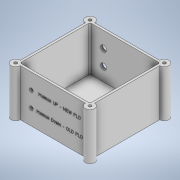
# Autodesk Inventor part: Case
Saved by Autodesk Inventor 2020 (Build 240168000, 168)
## iProperties
Created: 2019-12-06
Part Number: Case
Material: Generic
Document SubType Name: Modeling
Designer: Alex
Density: 1 g/cm^3
Appearance: Default
Author: Alex
Autodesk Inventor part; units mm, degrees
(part 1 of 2)
ref_plane "YZ Plane" through (0, 0, 0) normal (1, 0, 0) x (0, 1, 0)
ref_plane "XZ Plane" through (0, 0, 0) normal (0, 1, 0) x (-1, 0, 0)
ref_plane "XY Plane" through (0, 0, 0) normal (0, 0, 1) x (1, 0, 0)
sketch "Sketch1" plane through (0, 0, 0) normal (0, 1, 0) x (-1, 0, 0)
  line L0 (50, -50) -> (43.75, -50) construction
  line L1 (-50, -50) -> (-50, -43.75) construction
  line L2 (-50, 50) -> (-43.75, 50) construction
  line L3 (50, 50) -> (50, 43.75) construction
  arc A0 (43.75, -50) -> (50, -43.75) centre (50, -50) ccw
  arc A1 (-50, -43.75) -> (-43.75, -50) centre (-50, -50) ccw
  arc A2 (-43.75, 50) -> (-50, 43.75) centre (-50, 50) ccw
  arc A3 (50, 43.75) -> (43.75, 50) centre (50, 50) ccw
  line L4 (43.75, -50) -> (-43.75, -50)
  line L5 (50, -43.75) -> (50, -50) construction
  arc A4 (50, -43.75) -> (43.75, -50) centre (50, -50) ccw construction
  line L6 (50, 43.75) -> (50, -43.75)
  line L7 (43.75, 50) -> (50, 50) construction
  arc A5 (43.75, 50) -> (50, 43.75) centre (50, 50) ccw construction
  line L8 (-43.75, 50) -> (43.75, 50)
  line L9 (-50, 43.75) -> (-50, 50) construction
  arc A6 (-50, 43.75) -> (-43.75, 50) centre (-50, 50) ccw construction
  arc A7 (-43.75, -50) -> (-50, -43.75) centre (-50, -50) ccw construction
  line L10 (-43.75, -50) -> (-50, -50) construction
  line L11 (-50, -43.75) -> (-50, 43.75)
  point P0 (0, 0)
  point P1 (50, 0)
  point P2 (0, -50)
  dimension "d0" = 100
  dimension "d1" = 100
  dimension "d3" = 6.25
  constraints: 24 end point, 18 parallel, 16 point on circle, 9 perpendicular, 8 centre point, 4 coincident, 3 equal radius, 3 horizontal, 2 midpoint, 1 horizontal alignment, 1 vertical alignment
  measures "d0" distance of L1.start L0.start
  measures "d1" distance of L2.start L1.start
  measures "d3" radius of A0
extrude "Extrusion1" add sketch "Sketch1" along normal blind 3
sketch "Sketch2" plane through (0, 3, 0) normal (0, 1, 0) x (1, 0, 0)
  arc A0 (50, 43.75) -> (43.75, 50) centre (50, 50) ccw projected
  line L0 (43.75, 50) -> (-43.75, 50) projected
  arc A1 (-43.75, 50) -> (-50, 43.75) centre (-50, 50) ccw projected
  line L1 (-50, 43.75) -> (-50, -43.75) projected
  arc A2 (-50, -43.75) -> (-43.75, -50) centre (-50, -50) ccw projected
  line L2 (-43.75, -50) -> (43.75, -50) projected
  arc A3 (43.75, -50) -> (50, -43.75) centre (50, -50) ccw projected
  line L3 (50, -43.75) -> (50, 43.75) projected
  line L4 (-45, 47) -> (45, 47)
  line L5 (47, 45) -> (47, -45)
  line L6 (45, -47) -> (-45, -47)
  line L7 (-47, -45) -> (-47, 45)
  arc A4 (-45, 47) -> (-47, 45) centre (-45, 45) ccw
  arc A5 (-47, -45) -> (-45, -47) centre (-45, -45) ccw
  arc A6 (45, -47) -> (47, -45) centre (45, -45) ccw
  arc A7 (47, 45) -> (45, 47) centre (45, 45) ccw
  point P0 (0, 0)
  dimension "d6" = 3
  dimension "d7" = 2
  constraints: 8 end point, 8 point on circle, 8 tangent, 4 centre point, 3 equal radius, 3 other
  measures "d6" distance between parallel lines of L0 L4
  measures "d7" radius of A4
extrude "Extrusion2" add sketch "Sketch2" along normal blind 60
sketch "Sketch3" plane through (0, 63, 0) normal (0, 1, 0) x (1, 0, 0)
  arc A0 (-50, -43.75) -> (-43.75, -50) centre (-50, -50) ccw construction
  line L0 (-43.75, -50) -> (43.75, -50) construction
  arc A1 (43.75, -50) -> (50, -43.75) centre (50, -50) ccw construction
  line L1 (50, -43.75) -> (50, 43.75) construction
  arc A2 (50, 43.75) -> (43.75, 50) centre (50, 50) ccw construction
  line L2 (43.75, 50) -> (-43.75, 50) construction
  arc A3 (-43.75, 50) -> (-50, 43.75) centre (-50, 50) ccw construction
  line L3 (-50, 43.75) -> (-50, -43.75) construction
  line L4 (-45, 47) -> (45, 47) construction
  arc A4 (47, 45) -> (45, 47) centre (45, 45) ccw construction
  line L5 (47, 45) -> (47, -45) construction
  arc A5 (45, -47) -> (47, -45) centre (45, -45) ccw construction
  line L6 (45, -47) -> (-45, -47) construction
  arc A6 (-47, -45) -> (-45, -47) centre (-45, -45) ccw construction
  line L7 (-47, -45) -> (-47, 45) construction
  arc A7 (-45, 47) -> (-47, 45) centre (-45, 45) ccw construction
  point P0 (0, 0)
  constraints: 4 coincident
hole "Hole1" at (-50, 63, -50) at (50, 63, -50) at (50, 63, 50) at (-50, 63, 50) direction (0, -1, 0) diameter 4 depth 5
sketch "Sketch4" plane through (0, 3, 0) normal (0, 1, 0) x (1, 0, 0)
  line L0 (-9.3, 44) -> (44, 44) construction
  line L1 (44, 44) -> (44, -24.6) construction
  line L2 (44, -24.6) -> (-9.3, -24.6) construction
  line L3 (-9.3, -24.6) -> (-9.3, 44) construction
  arc A0 (-45, 47) -> (-47, 45) centre (-45, 45) ccw construction
  line L4 (-47, 45) -> (-47, -45) construction
  arc A1 (-47, -45) -> (-45, -47) centre (-45, -45) ccw construction
  line L5 (-45, -47) -> (45, -47) construction
  arc A2 (45, -47) -> (47, -45) centre (45, -45) ccw construction
  line L6 (47, -45) -> (47, 45) construction
  arc A3 (47, 45) -> (45, 47) centre (45, 45) ccw construction
  line L7 (45, 47) -> (-45, 47) construction
  line L8 (-4.2, -24.6) -> (0.8, -24.6)
  line L9 (0.8, -24.6) -> (0.8, -19.6)
  line L10 (0.8, -19.6) -> (-4.2, -19.6)
  line L11 (-4.2, -19.6) -> (-4.2, -24.6)
  line L12 (-4.2, -24.6) -> (0.8, -19.6) construction
  line L13 (0.8, -24.6) -> (-4.2, -19.6) construction
  line L14 (28.7, -24.6) -> (23.7, -24.6)
  line L15 (23.7, -24.6) -> (23.7, -19.6)
  line L16 (23.7, -19.6) -> (28.7, -19.6)
  line L17 (28.7, -19.6) -> (28.7, -24.6)
  line L18 (28.7, -24.6) -> (23.7, -19.6) construction
  line L19 (23.7, -24.6) -> (28.7, -19.6) construction
  line L20 (-8.3, 29) -> (13.7, 29)
  line L21 (13.7, 29) -> (13.7, 19)
  line L22 (13.7, 19) -> (-8.3, 19)
  line L23 (-8.3, 19) -> (-8.3, 29)
  line L24 (33, 37) -> (43, 37)
  line L25 (43, 37) -> (43, 32)
  line L26 (43, 32) -> (33, 32)
  line L27 (33, 32) -> (33, 37)
  point P0 (0, 0)
  point P1 (-6.8, 30)
  point P2 (41.4, 28.7)
  point P3 (-1.7, -22.1)
  point P4 (26.2, -22.1)
  dimension "d17" = 68.6
  dimension "d18" = 53.3
  dimension "d19" = 14
  dimension "d20" = 1.3
  dimension "d21" = 50.8
  dimension "d22" = 2.5
  dimension "d23" = 5.1
  dimension "d24" = 27.9
  dimension "d25" = 15.2
  dimension "d26" = 3
  dimension "d27" = 3
  dimension "d28" = 5
  dimension "d29" = 15
  dimension "d30" = 25
  dimension "d31" = 1
  dimension "d32" = 23
  dimension "d33" = 7
  dimension "d34" = 12
  dimension "d35" = 1
  dimension "d36" = 11
  constraints: 48 end point, 10 parallel, 5 horizontal, 5 perpendicular, 4 midpoint, 3 equal length, 1 horizontal alignment
  measures "d17" distance of L2.end L0.start
  measures "d18" distance of L0.start L0.end
  measures "d19" distance from line of point (-6.8, 30) L0
  measures "d20" vertical distance of point (41.4, 28.7) point (-6.8, 30)
  measures "d21" vertical distance of point (26.2, -22.1) point (41.4, 28.7)
  measures "d22" distance from line of point (-6.8, 30) L3
  measures "d23" horizontal distance of point (-1.7, -22.1) point (-6.8, 30)
  measures "d24" distance of point (26.2, -22.1) point (-1.7, -22.1)
  measures "d25" horizontal distance of point (41.4, 28.7) point (26.2, -22.1)
  measures "d26" distance between parallel lines of L0 L7
  measures "d27" distance between parallel lines of L6 L1
  measures "d28" distance of L9.end L10.end
  measures "d29" distance between parallel lines of L20 L0
  measures "d30" distance between parallel lines of L22 L0
  measures "d31" distance between parallel lines of L23 L3
  measures "d32" distance between parallel lines of L21 L3
  measures "d33" distance between parallel lines of L24 L0
  measures "d34" distance between parallel lines of L26 L0
  measures "d35" distance between parallel lines of L25 L1
  measures "d36" distance between parallel lines of L27 L1
extrude "Extrusion3" add sketch "Sketch4" along normal blind 3
chamfer "Chamfer1" distance 3 angle 45 16 edges at (2.7, 3, -19) (-8.3, 3, -24) (2.7, 3, -29) (13.7, 3, -24) (38, 3, -32) (33, 3, -34.5) (43, 3, -34.5) (38, 3, -37) (-4.2, 3, 22.1) (-1.7, 3, 19.6) (-1.7, 3, 24.6) (0.8, 3, 22.1) (26.2, 3, 24.6) (28.7, 3, 22.1) (23.7, 3, 22.1) (26.2, 3, 19.6)
sketch "Sketch5" plane through (0, 6, 0) normal (0, 1, 0) x (1, 0, 0)
  line L0 (0.8, -19.6) -> (-4.2, -19.6) projected
  line L1 (28.7, -19.6) -> (23.7, -19.6) projected
  line L2 (0.8, -24.6) -> (0.8, -19.6) projected
  point P0 (0, 0)
  point P1 (-1.7, -22.1)
  point P2 (26.2, -22.1)
  point P3 (-1.7, -19.6)
  point P4 (26.2, -19.6)
  point P5 (0.8, -22.1)
  point P6 (0.8, -22.1)
  constraints: 4 midpoint, 2 horizontal alignment, 2 vertical alignment
hole "Hole2" at (-1.7, 6, 22.1) at (26.2, 6, 22.1) direction (0, -1, 0) diameter 4 depth 5
sketch "Sketch6" plane through (-45, 3, -47) normal (0, 0, 1) x (1, 0, 0)
  line L0 (67.7, 15.6) -> (79.9, 15.6)
  line L1 (79.9, 15.6) -> (79.9, 4.6)
  line L2 (79.9, 4.6) -> (67.7, 4.6)
  line L3 (67.7, 4.6) -> (67.7, 15.6)
  line L4 (36.7, 3) -> (58.7, 3) construction
  line L5 (58.7, 3) -> (36.7, 3) construction
  line L6 (33.7, 0) -> (61.7, 0) construction
  line L7 (58.7, 3) -> (61.7, 0) construction
  line L8 (36.7, 3) -> (58.7, 3) construction
  line L9 (33.7, 0) -> (36.7, 3) construction
  line L10 (33.7, 0) -> (36.7, 3) construction
  line L11 (36.7, 3) -> (33.7, 0) construction
  line L12 (58.7, 3) -> (61.7, 0) construction
  line L13 (58.7, 3) -> (61.7, 0) construction
  line L14 (61.7, 0) -> (33.7, 0) construction
  line L15 (36.7, 3) -> (33.7, 0) construction
  line L16 (58.7, 3) -> (36.7, 3) construction
  line L17 (58.7, 3) -> (61.7, 0) construction
  point P0 (45, -3)
  point P1 (35.7, 0)
  point P2 (35.7, 0)
  point P3 (35.7, 0)
  point P4 (89, 0)
  point P5 (89, 0)
  point P6 (89, 0)
  dimension "d49" = 1.6
  dimension "d50" = 12.2
  dimension "d51" = 11
  dimension "d52" = 9.1
  constraints: 8 end point, 2 parallel, 1 horizontal, 1 perpendicular
  measures "d49" distance between parallel lines of L4 L2
  measures "d50" distance of L0.start L0.end
  measures "d51" distance of L2.end L0.start
  measures "d52" distance from line of L1 point (89, 0)
extrude "Extrusion4" cut sketch "Sketch6" against normal blind 3
sketch "Sketch7" plane through (43.75, 0, -50) normal (0, 0, -1) x (-1, 0, 0)
  line L0 (72.5, 42) -> (72.5, 63) construction
  line L1 (87.5, 63) -> (0, 63) construction
  line L2 (21.05, 7.6) -> (8.85, 7.6) construction
  line L3 (8.85, 7.6) -> (8.85, 18.6) construction
  line L4 (8.85, 18.6) -> (21.05, 18.6) construction
  line L5 (21.05, 18.6) -> (21.05, 7.6) construction
  line L6 (0, 0) -> (87.5, 0) construction
  line L7 (87.5, 0) -> (87.5, 63) construction
  line L8 (0, 63) -> (87.5, 63) construction
  line L9 (0, 0) -> (0, 63) construction
  line L10 (72.5, 42) -> (72.5, 21) construction
  line L11 (72.5, 21) -> (72.5, 0) construction
  line L12 (87.5, 0) -> (0, 0) construction
  point P0 (43.75, 0)
  dimension "d55" = 15
  constraints: 6 end point, 3 point on line, 2 collinear, 2 vertical, 1 vertical alignment
  measures "d55" distance between parallel lines of L7 L10
hole "Hole3" at (-28.75, 42, -50) at (-28.75, 21, -50) direction (0, 0, 1) diameter 8 depth 5
sketch "Sketch8" plane through (-43.75, 0, 50) normal (0, 0, 1) x (1, 0, 0)
  line L0 (0, 0) -> (87.5, 0) construction
  line L1 (87.5, 0) -> (87.5, 63) construction
  line L2 (0, 63) -> (87.5, 63) construction
  line L3 (0, 0) -> (0, 63) construction
  line L4 (15, 42) -> (15, 63) construction
  line L5 (15, 21) -> (15, 0) construction
  line L6 (87.5, 0) -> (0, 0) construction
  line L7 (15, 42) -> (15, 21) construction
  point P0 (43.75, 0)
  dimension "d63" = 15
  constraints: 6 end point, 3 vertical, 2 collinear, 2 point on line
  measures "d63" distance between parallel lines of L4 L3
hole "Hole4" at (-28.75, 42, 50) at (-28.75, 21, 50) direction (0, 0, -1) diameter 5 depth 5
sketch "Sketch9" plane through (-43.75, 0, 50) normal (0, 0, 1) x (1, 0, 0)
  line L0 (20.5, 47) -> (85.5, 47) construction
  line L1 (85.5, 47) -> (85.5, 37) construction
  line L2 (85.5, 37) -> (20.5, 37) construction
  line L3 (20.5, 37) -> (20.5, 47) construction
  line L4 (20.5, 26) -> (85.5, 26) construction
  line L5 (85.5, 26) -> (85.5, 16) construction
  line L6 (85.5, 16) -> (20.5, 16) construction
  line L7 (20.5, 16) -> (20.5, 26) construction
  circle A0 centre (15, 42) radius 2.5 construction
  circle A1 centre (15, 21) radius 2.5 construction
  line L8 (0, 0) -> (87.5, 0) construction
  line L9 (87.5, 0) -> (87.5, 63) construction
  line L10 (0, 63) -> (87.5, 63) construction
  line L11 (0, 0) -> (0, 63) construction
  spline S0 degree 2 poles (28.025, 40.2168) (28.025, 40.0318) (27.8491, 40.0318) knots 0 0 0 1 1 1
  spline S1 degree 2 poles (27.8491, 40.0318) (27.6702, 40.0318) (27.6702, 40.2168) knots 0 0 0 1 1 1
  line L12 (27.6702, 40.2168) -> (27.6702, 43.3859)
  line L13 (27.6702, 43.3859) -> (26.627, 41.8757)
  spline S2 degree 2 poles (26.627, 41.8757) (26.533, 41.7422) (26.4117, 41.7422) knots 0 0 0 1 1 1
  spline S3 degree 2 poles (26.4117, 41.7422) (26.2964, 41.7422) (26.2146, 41.8605) knots 0 0 0 1 1 1
  line L14 (26.2146, 41.8605) -> (25.1713, 43.398)
  line L15 (25.1713, 43.398) -> (25.1713, 40.2168)
  spline S4 degree 2 poles (25.1713, 40.2168) (25.1713, 40.0318) (24.9924, 40.0318) knots 0 0 0 1 1 1
  spline S5 degree 2 poles (24.9924, 40.0318) (24.8105, 40.0318) (24.8105, 40.2168) knots 0 0 0 1 1 1
  line L16 (24.8105, 40.2168) -> (24.8105, 43.8105)
  spline S6 degree 2 poles (24.8105, 43.8105) (24.8105, 44.0076) (25.0076, 44.0076) knots 0 0 0 1 1 1
  spline S7 degree 2 poles (25.0076, 44.0076) (25.1744, 44.0076) (25.2866, 43.8499) knots 0 0 0 1 1 1
  line L17 (25.2866, 43.8499) -> (26.4177, 42.2244)
  line L18 (26.4177, 42.2244) -> (27.5519, 43.8469)
  spline S8 degree 2 poles (27.5519, 43.8469) (27.6823, 44.0318) (27.834, 44.0318) knots 0 0 0 1 1 1
  spline S9 degree 2 poles (27.834, 44.0318) (28.025, 44.0318) (28.025, 43.8105) knots 0 0 0 1 1 1
  line L19 (28.025, 43.8105) -> (28.025, 40.2168)
  spline S10 degree 2 poles (29.514, 40.2229) (29.514, 40.0379) (29.3351, 40.0379) knots 0 0 0 1 1 1
  spline S11 degree 2 poles (29.3351, 40.0379) (29.1531, 40.0379) (29.1531, 40.2229) knots 0 0 0 1 1 1
  line L20 (29.1531, 40.2229) -> (29.1531, 43.119)
  spline S12 degree 2 poles (29.1531, 43.119) (29.1531, 43.304) (29.3351, 43.304) knots 0 0 0 1 1 1
  spline S13 degree 2 poles (29.3351, 43.304) (29.514, 43.304) (29.514, 43.119) knots 0 0 0 1 1 1
  line L21 (29.514, 43.119) -> (29.514, 40.2229)
  spline S14 degree 2 poles (32.7559, 42.4003) (32.7559, 41.9181) (32.4375, 41.6725) knots 0 0 0 1 1 1
  spline S15 degree 2 poles (32.4375, 41.6725) (32.2252, 41.5057) (32.0159, 41.5057) knots 0 0 0 1 1 1
  line L22 (32.0159, 41.5057) -> (31.9219, 41.5087)
  line L23 (31.9219, 41.5087) -> (32.7225, 40.323)
  spline S16 degree 2 poles (32.7225, 40.323) (32.7559, 40.2684) (32.7559, 40.2168) knots 0 0 0 1 1 1
  spline S17 degree 2 poles (32.7559, 40.2168) (32.7559, 40.141) (32.6467, 40.0318) (32.577, 40.0318) knots 0 0 0 1 2 2 2
  spline S18 degree 2 poles (32.577, 40.0318) (32.4951, 40.0318) (32.4435, 40.1077) knots 0 0 0 1 1 1
  line L24 (32.4435, 40.1077) -> (31.4913, 41.5057)
  line L25 (31.4913, 41.5057) -> (30.8241, 41.5057)
  line L26 (30.8241, 41.5057) -> (30.8241, 40.2168)
  spline S19 degree 2 poles (30.8241, 40.2168) (30.8241, 40.0318) (30.6513, 40.0318) knots 0 0 0 1 1 1
  spline S20 degree 2 poles (30.6513, 40.0318) (30.4754, 40.0318) (30.4754, 40.2168) knots 0 0 0 1 1 1
  line L27 (30.4754, 40.2168) -> (30.4754, 43.298)
  line L28 (30.4754, 43.298) -> (31.84, 43.298)
  spline S21 degree 2 poles (31.84, 43.298) (32.2221, 43.298) (32.4769, 43.0705) knots 0 0 0 1 1 1
  spline S22 degree 2 poles (32.4769, 43.0705) (32.7559, 42.8218) (32.7559, 42.4003) knots 0 0 0 1 1 1
  spline S23 degree 2 poles (32.4071, 42.4003) (32.4071, 42.6581) (32.0766, 42.9371) (31.84, 42.9371) knots 0 0 0 1 2 2 2
  line L29 (31.84, 42.9371) -> (30.8241, 42.9371)
  line L30 (30.8241, 42.9371) -> (30.8241, 41.8666)
  line L31 (30.8241, 41.8666) -> (32.0129, 41.8666)
  spline S24 degree 2 poles (32.0129, 41.8666) (32.1221, 41.8666) (32.2434, 41.9757) knots 0 0 0 1 1 1
  spline S25 degree 2 poles (32.2434, 41.9757) (32.4071, 42.1274) (32.4071, 42.4003) knots 0 0 0 1 1 1
  spline S26 degree 2 poles (35.6187, 42.4003) (35.6187, 41.9181) (35.3002, 41.6725) knots 0 0 0 1 1 1
  spline S27 degree 2 poles (35.3002, 41.6725) (35.0879, 41.5057) (34.8787, 41.5057) knots 0 0 0 1 1 1
  line L32 (34.8787, 41.5057) -> (34.7847, 41.5087)
  line L33 (34.7847, 41.5087) -> (35.5853, 40.323)
  spline S28 degree 2 poles (35.5853, 40.323) (35.6187, 40.2684) (35.6187, 40.2168) knots 0 0 0 1 1 1
  spline S29 degree 2 poles (35.6187, 40.2168) (35.6187, 40.141) (35.5095, 40.0318) (35.4397, 40.0318) knots 0 0 0 1 2 2 2
  spline S30 degree 2 poles (35.4397, 40.0318) (35.3578, 40.0318) (35.3063, 40.1077) knots 0 0 0 1 1 1
  line L34 (35.3063, 40.1077) -> (34.3541, 41.5057)
  line L35 (34.3541, 41.5057) -> (33.6869, 41.5057)
  line L36 (33.6869, 41.5057) -> (33.6869, 40.2168)
  spline S31 degree 2 poles (33.6869, 40.2168) (33.6869, 40.0318) (33.514, 40.0318) knots 0 0 0 1 1 1
  spline S32 degree 2 poles (33.514, 40.0318) (33.3381, 40.0318) (33.3381, 40.2168) knots 0 0 0 1 1 1
  line L37 (33.3381, 40.2168) -> (33.3381, 43.298)
  line L38 (33.3381, 43.298) -> (34.7028, 43.298)
  spline S33 degree 2 poles (34.7028, 43.298) (35.0849, 43.298) (35.3397, 43.0705) knots 0 0 0 1 1 1
  spline S34 degree 2 poles (35.3397, 43.0705) (35.6187, 42.8218) (35.6187, 42.4003) knots 0 0 0 1 1 1
  spline S35 degree 2 poles (35.2699, 42.4003) (35.2699, 42.6581) (34.9393, 42.9371) (34.7028, 42.9371) knots 0 0 0 1 2 2 2
  line L39 (34.7028, 42.9371) -> (33.6869, 42.9371)
  line L40 (33.6869, 42.9371) -> (33.6869, 41.8666)
  line L41 (33.6869, 41.8666) -> (34.8757, 41.8666)
  spline S36 degree 2 poles (34.8757, 41.8666) (34.9848, 41.8666) (35.1061, 41.9757) knots 0 0 0 1 1 1
  spline S37 degree 2 poles (35.1061, 41.9757) (35.2699, 42.1274) (35.2699, 42.4003) knots 0 0 0 1 1 1
  spline S38 degree 2 poles (38.5299, 41.6694) (38.5299, 41.0296) (38.2115, 40.5534) knots 0 0 0 1 1 1
  spline S39 degree 2 poles (38.2115, 40.5534) (37.8628, 40.0379) (37.323, 40.0379) knots 0 0 0 1 1 1
  spline S40 degree 2 poles (37.323, 40.0379) (36.7832, 40.0379) (36.4344, 40.5595) knots 0 0 0 1 1 1
  spline S41 degree 2 poles (36.4344, 40.5595) (36.116, 41.0356) (36.116, 41.6694) knots 0 0 0 1 1 1
  spline S42 degree 2 poles (36.116, 41.6694) (36.116, 42.2972) (36.4405, 42.7794) knots 0 0 0 1 1 1
  spline S43 degree 2 poles (36.4405, 42.7794) (36.7953, 43.2889) (37.323, 43.2889) knots 0 0 0 1 1 1
  spline S44 degree 2 poles (37.323, 43.2889) (37.887, 43.2889) (38.2237, 42.7733) knots 0 0 0 1 1 1
  spline S45 degree 2 poles (38.2237, 42.7733) (38.5299, 42.3063) (38.5299, 41.6694) knots 0 0 0 1 1 1
  spline S46 degree 2 poles (38.1812, 41.6694) (38.1812, 42.1668) (37.978, 42.5155) knots 0 0 0 1 1 1
  spline S47 degree 2 poles (37.978, 42.5155) (37.7475, 42.928) (37.323, 42.928) knots 0 0 0 1 1 1
  spline S48 degree 2 poles (37.323, 42.928) (36.9227, 42.928) (36.6801, 42.5155) knots 0 0 0 1 1 1
  spline S49 degree 2 poles (36.6801, 42.5155) (36.4647, 42.1577) (36.4647, 41.6694) knots 0 0 0 1 1 1
  spline S50 degree 2 poles (36.4647, 41.6694) (36.4647, 41.1691) (36.674, 40.8112) knots 0 0 0 1 1 1
  spline S51 degree 2 poles (36.674, 40.8112) (36.9105, 40.3988) (37.323, 40.3988) knots 0 0 0 1 1 1
  spline S52 degree 2 poles (37.323, 40.3988) (37.7354, 40.3988) (37.9719, 40.8112) knots 0 0 0 1 1 1
  spline S53 degree 2 poles (37.9719, 40.8112) (38.1812, 41.1691) (38.1812, 41.6694) knots 0 0 0 1 1 1
  spline S54 degree 2 poles (41.4473, 42.4003) (41.4473, 41.9181) (41.1289, 41.6725) knots 0 0 0 1 1 1
  spline S55 degree 2 poles (41.1289, 41.6725) (40.9166, 41.5057) (40.7074, 41.5057) knots 0 0 0 1 1 1
  line L42 (40.7074, 41.5057) -> (40.6133, 41.5087)
  line L43 (40.6133, 41.5087) -> (41.414, 40.323)
  spline S56 degree 2 poles (41.414, 40.323) (41.4473, 40.2684) (41.4473, 40.2168) knots 0 0 0 1 1 1
  spline S57 degree 2 poles (41.4473, 40.2168) (41.4473, 40.141) (41.3381, 40.0318) (41.2684, 40.0318) knots 0 0 0 1 2 2 2
  spline S58 degree 2 poles (41.2684, 40.0318) (41.1865, 40.0318) (41.135, 40.1077) knots 0 0 0 1 1 1
  line L44 (41.135, 40.1077) -> (40.1827, 41.5057)
  line L45 (40.1827, 41.5057) -> (39.5155, 41.5057)
  line L46 (39.5155, 41.5057) -> (39.5155, 40.2168)
  spline S59 degree 2 poles (39.5155, 40.2168) (39.5155, 40.0318) (39.3427, 40.0318) knots 0 0 0 1 1 1
  spline S60 degree 2 poles (39.3427, 40.0318) (39.1668, 40.0318) (39.1668, 40.2168) knots 0 0 0 1 1 1
  line L47 (39.1668, 40.2168) -> (39.1668, 43.298)
  line L48 (39.1668, 43.298) -> (40.5315, 43.298)
  spline S61 degree 2 poles (40.5315, 43.298) (40.9136, 43.298) (41.1683, 43.0705) knots 0 0 0 1 1 1
  spline S62 degree 2 poles (41.1683, 43.0705) (41.4473, 42.8218) (41.4473, 42.4003) knots 0 0 0 1 1 1
  spline S63 degree 2 poles (41.0986, 42.4003) (41.0986, 42.6581) (40.768, 42.9371) (40.5315, 42.9371) knots 0 0 0 1 2 2 2
  line L49 (40.5315, 42.9371) -> (39.5155, 42.9371)
  line L50 (39.5155, 42.9371) -> (39.5155, 41.8666)
  line L51 (39.5155, 41.8666) -> (40.7043, 41.8666)
  spline S64 degree 2 poles (40.7043, 41.8666) (40.8135, 41.8666) (40.9348, 41.9757) knots 0 0 0 1 1 1
  spline S65 degree 2 poles (40.9348, 41.9757) (41.0986, 42.1274) (41.0986, 42.4003) knots 0 0 0 1 1 1
  spline S66 degree 2 poles (47.0455, 41.3419) (47.0455, 40.1077) (45.7354, 40.0076) knots 0 0 0 1 1 1
  spline S67 degree 2 poles (45.7354, 40.0076) (45.1895, 39.9682) (44.765, 40.2926) knots 0 0 0 1 1 1
  spline S68 degree 2 poles (44.765, 40.2926) (44.2889, 40.6626) (44.2889, 41.3086) knots 0 0 0 1 1 1
  line L52 (44.2889, 41.3086) -> (44.2889, 43.8408)
  spline S69 degree 2 poles (44.2889, 43.8408) (44.2889, 44.0258) (44.4678, 44.0258) knots 0 0 0 1 1 1
  spline S70 degree 2 poles (44.4678, 44.0258) (44.6437, 44.0258) (44.6437, 43.8408) knots 0 0 0 1 1 1
  line L53 (44.6437, 43.8408) -> (44.6437, 41.3086)
  spline S71 degree 2 poles (44.6437, 41.3086) (44.6437, 40.8446) (44.9985, 40.5716) knots 0 0 0 1 1 1
  spline S72 degree 2 poles (44.9985, 40.5716) (45.3108, 40.3321) (45.7111, 40.3624) knots 0 0 0 1 1 1
  spline S73 degree 2 poles (45.7111, 40.3624) (46.6907, 40.4261) (46.6907, 41.345) knots 0 0 0 1 1 1
  line L54 (46.6907, 41.345) -> (46.6907, 43.8408)
  spline S74 degree 2 poles (46.6907, 43.8408) (46.6907, 44.0258) (46.8696, 44.0258) knots 0 0 0 1 1 1
  spline S75 degree 2 poles (46.8696, 44.0258) (47.0455, 44.0258) (47.0455, 43.8408) knots 0 0 0 1 1 1
  line L55 (47.0455, 43.8408) -> (47.0455, 41.3419)
  spline S76 degree 2 poles (50.257, 42.9917) (50.257, 42.5489) (50.0235, 42.2881) knots 0 0 0 1 1 1
  spline S77 degree 2 poles (50.0235, 42.2881) (49.7809, 42.0091) (49.3442, 42.0091) knots 0 0 0 1 1 1
  line L56 (49.3442, 42.0091) -> (48.0796, 42.0091)
  line L57 (48.0796, 42.0091) -> (48.0796, 40.2168)
  spline S78 degree 2 poles (48.0796, 40.2168) (48.0796, 40.0318) (47.9037, 40.0318) knots 0 0 0 1 1 1
  spline S79 degree 2 poles (47.9037, 40.0318) (47.7248, 40.0318) (47.7248, 40.2168) knots 0 0 0 1 1 1
  line L58 (47.7248, 40.2168) -> (47.7248, 44.0197)
  line L59 (47.7248, 44.0197) -> (49.2472, 44.0197)
  spline S80 degree 2 poles (49.2472, 44.0197) (49.7566, 44.0197) (50.0174, 43.7286) knots 0 0 0 1 1 1
  spline S81 degree 2 poles (50.0174, 43.7286) (50.257, 43.4617) (50.257, 42.9917) knots 0 0 0 1 1 1
  spline S82 degree 2 poles (49.9022, 42.9917) (49.9022, 43.6588) (49.2472, 43.6588) knots 0 0 0 1 1 1
  line L60 (49.2472, 43.6588) -> (48.0796, 43.6588)
  line L61 (48.0796, 43.6588) -> (48.0796, 42.376)
  line L62 (48.0796, 42.376) -> (49.3442, 42.376)
  spline S83 degree 2 poles (49.3442, 42.376) (49.6111, 42.376) (49.9022, 42.7127) (49.9022, 42.9917) knots 0 0 0 1 2 2 2
  line L63 (54.7968, 41.4996) -> (53.3563, 41.4996)
  spline S84 degree 2 poles (53.3563, 41.4996) (53.1774, 41.4996) (53.1774, 41.6785) knots 0 0 0 1 1 1
  spline S85 degree 2 poles (53.1774, 41.6785) (53.1774, 41.8544) (53.3563, 41.8544) knots 0 0 0 1 1 1
  line L64 (53.3563, 41.8544) -> (54.7968, 41.8544)
  spline S86 degree 2 poles (54.7968, 41.8544) (54.9757, 41.8544) (54.9757, 41.6785) knots 0 0 0 1 1 1
  spline S87 degree 2 poles (54.9757, 41.6785) (54.9757, 41.4996) (54.7968, 41.4996) knots 0 0 0 1 1 1
  spline S88 degree 2 poles (60.7346, 40.2077) (60.7346, 40.0318) (60.5951, 40.0318) knots 0 0 0 1 1 1
  spline S89 degree 2 poles (60.5951, 40.0318) (60.4829, 40.0318) (60.3889, 40.1622) knots 0 0 0 1 1 1
  line L65 (60.3889, 40.1622) -> (58.2115, 43.3071)
  line L66 (58.2115, 43.3071) -> (58.2115, 40.2168)
  spline S90 degree 2 poles (58.2115, 40.2168) (58.2115, 40.0318) (58.0326, 40.0318) knots 0 0 0 1 1 1
  spline S91 degree 2 poles (58.0326, 40.0318) (57.8506, 40.0318) (57.8506, 40.2168) knots 0 0 0 1 1 1
  line L67 (57.8506, 40.2168) -> (57.8506, 43.862)
  spline S92 degree 2 poles (57.8506, 43.862) (57.8506, 44.0318) (58.0083, 44.0318) knots 0 0 0 1 1 1
  spline S93 degree 2 poles (58.0083, 44.0318) (58.1296, 44.0318) (58.2237, 43.8984) knots 0 0 0 1 1 1
  line L68 (58.2237, 43.8984) -> (60.3798, 40.8021)
  line L69 (60.3798, 40.8021) -> (60.3798, 43.8469)
  spline S94 degree 2 poles (60.3798, 43.8469) (60.3798, 44.0318) (60.5588, 44.0318) knots 0 0 0 1 1 1
  spline S95 degree 2 poles (60.5588, 44.0318) (60.7346, 44.0318) (60.7346, 43.8469) knots 0 0 0 1 1 1
  line L70 (60.7346, 43.8469) -> (60.7346, 40.2077)
  line L71 (64.0159, 40.0895) -> (61.5838, 40.0895)
  line L72 (61.5838, 40.0895) -> (61.5838, 44.0197)
  line L73 (61.5838, 44.0197) -> (64.0159, 44.0197)
  spline S96 degree 2 poles (64.0159, 44.0197) (64.1948, 44.0197) (64.1948, 43.8378) knots 0 0 0 1 1 1
  spline S97 degree 2 poles (64.1948, 43.8378) (64.1948, 43.6528) (64.0159, 43.6528) knots 0 0 0 1 1 1
  line L74 (64.0159, 43.6528) -> (61.9386, 43.6528)
  line L75 (61.9386, 43.6528) -> (61.9386, 42.4276)
  line L76 (61.9386, 42.4276) -> (63.8946, 42.4276)
  spline S98 degree 2 poles (63.8946, 42.4276) (64.0796, 42.4276) (64.0796, 42.2487) knots 0 0 0 1 1 1
  spline S99 degree 2 poles (64.0796, 42.2487) (64.0796, 42.0667) (63.8946, 42.0667) knots 0 0 0 1 1 1
  line L77 (63.8946, 42.0667) -> (61.9386, 42.0667)
  line L78 (61.9386, 42.0667) -> (61.9386, 40.4503)
  line L79 (61.9386, 40.4503) -> (64.0159, 40.4503)
  spline S100 degree 2 poles (64.0159, 40.4503) (64.1948, 40.4503) (64.1948, 40.2714) knots 0 0 0 1 1 1
  spline S101 degree 2 poles (64.1948, 40.2714) (64.1948, 40.0895) (64.0159, 40.0895) knots 0 0 0 1 1 1
  line L80 (68.9257, 43.8044) -> (68.2312, 40.2047)
  spline S102 degree 2 poles (68.2312, 40.2047) (68.1948, 40.0258) (68.0068, 40.0258) knots 0 0 0 1 1 1
  spline S103 degree 2 poles (68.0068, 40.0258) (67.8097, 40.0258) (67.7582, 40.2047) knots 0 0 0 1 1 1
  line L81 (67.7582, 40.2047) -> (66.9363, 43.1736)
  line L82 (66.9363, 43.1736) -> (66.1812, 40.2047)
  spline S104 degree 2 poles (66.1812, 40.2047) (66.1357, 40.0258) (65.9356, 40.0258) knots 0 0 0 1 1 1
  spline S105 degree 2 poles (65.9356, 40.0258) (65.7324, 40.0258) (65.699, 40.2047) knots 0 0 0 1 1 1
  line L83 (65.699, 40.2047) -> (64.956, 43.8044)
  spline S106 degree 2 poles (64.956, 43.8044) (64.9378, 43.9045) (65.0561, 44.0197) (65.135, 44.0197) knots 0 0 0 1 2 2 2
  spline S107 degree 2 poles (65.135, 44.0197) (65.2866, 44.0197) (65.3169, 43.8741) knots 0 0 0 1 1 1
  line L84 (65.3169, 43.8741) -> (65.9598, 40.7566)
  line L85 (65.9598, 40.7566) -> (66.7483, 43.8863)
  spline S108 degree 2 poles (66.7483, 43.8863) (66.7847, 44.0197) (66.9242, 44.0197) knots 0 0 0 1 1 1
  spline S109 degree 2 poles (66.9242, 44.0197) (67.0698, 44.0197) (67.1031, 43.8863) knots 0 0 0 1 1 1
  line L86 (67.1031, 43.8863) -> (67.9613, 40.7839)
  line L87 (67.9613, 40.7839) -> (68.5648, 43.8741)
  spline S110 degree 2 poles (68.5648, 43.8741) (68.5951, 44.0197) (68.7407, 44.0197) knots 0 0 0 1 1 1
  spline S111 degree 2 poles (68.7407, 44.0197) (68.8287, 44.0197) (68.9439, 43.9045) (68.9257, 43.8044) knots 0 0 0 1 2 2 2
  spline S112 degree 2 poles (74.4117, 42.9917) (74.4117, 42.5489) (74.1782, 42.2881) knots 0 0 0 1 1 1
  spline S113 degree 2 poles (74.1782, 42.2881) (73.9356, 42.0091) (73.4989, 42.0091) knots 0 0 0 1 1 1
  line L88 (73.4989, 42.0091) -> (72.2343, 42.0091)
  line L89 (72.2343, 42.0091) -> (72.2343, 40.2168)
  spline S114 degree 2 poles (72.2343, 40.2168) (72.2343, 40.0318) (72.0584, 40.0318) knots 0 0 0 1 1 1
  spline S115 degree 2 poles (72.0584, 40.0318) (71.8795, 40.0318) (71.8795, 40.2168) knots 0 0 0 1 1 1
  line L90 (71.8795, 40.2168) -> (71.8795, 44.0197)
  line L91 (71.8795, 44.0197) -> (73.4018, 44.0197)
  spline S116 degree 2 poles (73.4018, 44.0197) (73.9113, 44.0197) (74.1721, 43.7286) knots 0 0 0 1 1 1
  spline S117 degree 2 poles (74.1721, 43.7286) (74.4117, 43.4617) (74.4117, 42.9917) knots 0 0 0 1 1 1
  spline S118 degree 2 poles (74.0569, 42.9917) (74.0569, 43.6588) (73.4018, 43.6588) knots 0 0 0 1 1 1
  line L92 (73.4018, 43.6588) -> (72.2343, 43.6588)
  line L93 (72.2343, 43.6588) -> (72.2343, 42.376)
  line L94 (72.2343, 42.376) -> (73.4989, 42.376)
  spline S119 degree 2 poles (73.4989, 42.376) (73.7657, 42.376) (74.0569, 42.7127) (74.0569, 42.9917) knots 0 0 0 1 2 2 2
  line L95 (77.5322, 40.0834) -> (75.1001, 40.0834)
  line L96 (75.1001, 40.0834) -> (75.1001, 43.8347)
  spline S120 degree 2 poles (75.1001, 43.8347) (75.1001, 44.0197) (75.279, 44.0197) knots 0 0 0 1 1 1
  spline S121 degree 2 poles (75.279, 44.0197) (75.4549, 44.0197) (75.4549, 43.8347) knots 0 0 0 1 1 1
  line L97 (75.4549, 43.8347) -> (75.4549, 40.4443)
  line L98 (75.4549, 40.4443) -> (77.5322, 40.4443)
  spline S122 degree 2 poles (77.5322, 40.4443) (77.7111, 40.4443) (77.7111, 40.2654) knots 0 0 0 1 1 1
  spline S123 degree 2 poles (77.7111, 40.2654) (77.7111, 40.0834) (77.5322, 40.0834) knots 0 0 0 1 1 1
  spline S124 degree 2 poles (81.1016, 42.1729) (81.1016, 41.0993) (80.5375, 40.5413) knots 0 0 0 1 1 1
  spline S125 degree 2 poles (80.5375, 40.5413) (80.0735, 40.0895) (79.4124, 40.0895) knots 0 0 0 1 1 1
  line L99 (79.4124, 40.0895) -> (78.3965, 40.0895)
  line L100 (78.3965, 40.0895) -> (78.3965, 44.0197)
  line L101 (78.3965, 44.0197) -> (79.4064, 44.0197)
  spline S126 degree 2 poles (79.4064, 44.0197) (80.0614, 44.0197) (80.5375, 43.5891) knots 0 0 0 1 1 1
  spline S127 degree 2 poles (80.5375, 43.5891) (81.1016, 43.0796) (81.1016, 42.1729) knots 0 0 0 1 1 1
  spline S128 degree 2 poles (80.7468, 42.1759) (80.7468, 42.8946) (80.301, 43.3071) knots 0 0 0 1 1 1
  spline S129 degree 2 poles (80.301, 43.3071) (79.9219, 43.6497) (79.4064, 43.6497) knots 0 0 0 1 1 1
  line L102 (79.4064, 43.6497) -> (78.7513, 43.6497)
  line L103 (78.7513, 43.6497) -> (78.7513, 40.4503)
  line L104 (78.7513, 40.4503) -> (79.4124, 40.4503)
  spline S130 degree 2 poles (79.4124, 40.4503) (79.9401, 40.4503) (80.3071, 40.8324) knots 0 0 0 1 1 1
  spline S131 degree 2 poles (80.3071, 40.8324) (80.7468, 41.2934) (80.7468, 42.1759) knots 0 0 0 1 1 1
  spline S132 degree 2 poles (25.4246, 19.1865) (25.4246, 19.0015) (25.2487, 19.0015) knots 0 0 0 1 1 1
  spline S133 degree 2 poles (25.2487, 19.0015) (25.0697, 19.0015) (25.0697, 19.1865) knots 0 0 0 1 1 1
  line L105 (25.0697, 19.1865) -> (25.0697, 22.3556)
  line L106 (25.0697, 22.3556) -> (24.0265, 20.8453)
  spline S134 degree 2 poles (24.0265, 20.8453) (23.9325, 20.7119) (23.8112, 20.7119) knots 0 0 0 1 1 1
  spline S135 degree 2 poles (23.8112, 20.7119) (23.696, 20.7119) (23.6141, 20.8302) knots 0 0 0 1 1 1
  line L107 (23.6141, 20.8302) -> (22.5709, 22.3677)
  line L108 (22.5709, 22.3677) -> (22.5709, 19.1865)
  spline S136 degree 2 poles (22.5709, 19.1865) (22.5709, 19.0015) (22.392, 19.0015) knots 0 0 0 1 1 1
  spline S137 degree 2 poles (22.392, 19.0015) (22.21, 19.0015) (22.21, 19.1865) knots 0 0 0 1 1 1
  line L109 (22.21, 19.1865) -> (22.21, 22.7801)
  spline S138 degree 2 poles (22.21, 22.7801) (22.21, 22.9773) (22.4071, 22.9773) knots 0 0 0 1 1 1
  spline S139 degree 2 poles (22.4071, 22.9773) (22.5739, 22.9773) (22.6861, 22.8196) knots 0 0 0 1 1 1
  line L110 (22.6861, 22.8196) -> (23.8173, 21.1941)
  line L111 (23.8173, 21.1941) -> (24.9515, 22.8165)
  spline S140 degree 2 poles (24.9515, 22.8165) (25.0819, 23.0015) (25.2335, 23.0015) knots 0 0 0 1 1 1
  spline S141 degree 2 poles (25.2335, 23.0015) (25.4246, 23.0015) (25.4246, 22.7801) knots 0 0 0 1 1 1
  line L112 (25.4246, 22.7801) -> (25.4246, 19.1865)
  spline S142 degree 2 poles (26.9136, 19.1926) (26.9136, 19.0076) (26.7346, 19.0076) knots 0 0 0 1 1 1
  spline S143 degree 2 poles (26.7346, 19.0076) (26.5527, 19.0076) (26.5527, 19.1926) knots 0 0 0 1 1 1
  line L113 (26.5527, 19.1926) -> (26.5527, 22.0887)
  spline S144 degree 2 poles (26.5527, 22.0887) (26.5527, 22.2737) (26.7346, 22.2737) knots 0 0 0 1 1 1
  spline S145 degree 2 poles (26.7346, 22.2737) (26.9136, 22.2737) (26.9136, 22.0887) knots 0 0 0 1 1 1
  line L114 (26.9136, 22.0887) -> (26.9136, 19.1926)
  spline S146 degree 2 poles (30.1554, 21.37) (30.1554, 20.8878) (29.837, 20.6422) knots 0 0 0 1 1 1
  spline S147 degree 2 poles (29.837, 20.6422) (29.6247, 20.4754) (29.4155, 20.4754) knots 0 0 0 1 1 1
  line L115 (29.4155, 20.4754) -> (29.3215, 20.4784)
  line L116 (29.3215, 20.4784) -> (30.1221, 19.2926)
  spline S148 degree 2 poles (30.1221, 19.2926) (30.1554, 19.2381) (30.1554, 19.1865) knots 0 0 0 1 1 1
  spline S149 degree 2 poles (30.1554, 19.1865) (30.1554, 19.1107) (30.0462, 19.0015) (29.9765, 19.0015) knots 0 0 0 1 2 2 2
  spline S150 degree 2 poles (29.9765, 19.0015) (29.8946, 19.0015) (29.8431, 19.0773) knots 0 0 0 1 1 1
  line L117 (29.8431, 19.0773) -> (28.8908, 20.4754)
  line L118 (28.8908, 20.4754) -> (28.2237, 20.4754)
  line L119 (28.2237, 20.4754) -> (28.2237, 19.1865)
  spline S151 degree 2 poles (28.2237, 19.1865) (28.2237, 19.0015) (28.0508, 19.0015) knots 0 0 0 1 1 1
  spline S152 degree 2 poles (28.0508, 19.0015) (27.8749, 19.0015) (27.8749, 19.1865) knots 0 0 0 1 1 1
  line L120 (27.8749, 19.1865) -> (27.8749, 22.2676)
  line L121 (27.8749, 22.2676) -> (29.2396, 22.2676)
  spline S153 degree 2 poles (29.2396, 22.2676) (29.6217, 22.2676) (29.8764, 22.0402) knots 0 0 0 1 1 1
  spline S154 degree 2 poles (29.8764, 22.0402) (30.1554, 21.7915) (30.1554, 21.37) knots 0 0 0 1 1 1
  spline S155 degree 2 poles (29.8067, 21.37) (29.8067, 21.6277) (29.4761, 21.9067) (29.2396, 21.9067) knots 0 0 0 1 2 2 2
  line L122 (29.2396, 21.9067) -> (28.2237, 21.9067)
  line L123 (28.2237, 21.9067) -> (28.2237, 20.8362)
  line L124 (28.2237, 20.8362) -> (29.4124, 20.8362)
  spline S156 degree 2 poles (29.4124, 20.8362) (29.5216, 20.8362) (29.6429, 20.9454) knots 0 0 0 1 1 1
  spline S157 degree 2 poles (29.6429, 20.9454) (29.8067, 21.097) (29.8067, 21.37) knots 0 0 0 1 1 1
  spline S158 degree 2 poles (33.0182, 21.37) (33.0182, 20.8878) (32.6998, 20.6422) knots 0 0 0 1 1 1
  spline S159 degree 2 poles (32.6998, 20.6422) (32.4875, 20.4754) (32.2782, 20.4754) knots 0 0 0 1 1 1
  line L125 (32.2782, 20.4754) -> (32.1842, 20.4784)
  line L126 (32.1842, 20.4784) -> (32.9848, 19.2926)
  spline S160 degree 2 poles (32.9848, 19.2926) (33.0182, 19.2381) (33.0182, 19.1865) knots 0 0 0 1 1 1
  spline S161 degree 2 poles (33.0182, 19.1865) (33.0182, 19.1107) (32.909, 19.0015) (32.8393, 19.0015) knots 0 0 0 1 2 2 2
  spline S162 degree 2 poles (32.8393, 19.0015) (32.7574, 19.0015) (32.7058, 19.0773) knots 0 0 0 1 1 1
  line L127 (32.7058, 19.0773) -> (31.7536, 20.4754)
  line L128 (31.7536, 20.4754) -> (31.0864, 20.4754)
  line L129 (31.0864, 20.4754) -> (31.0864, 19.1865)
  spline S163 degree 2 poles (31.0864, 19.1865) (31.0864, 19.0015) (30.9136, 19.0015) knots 0 0 0 1 1 1
  spline S164 degree 2 poles (30.9136, 19.0015) (30.7377, 19.0015) (30.7377, 19.1865) knots 0 0 0 1 1 1
  line L130 (30.7377, 19.1865) -> (30.7377, 22.2676)
  line L131 (30.7377, 22.2676) -> (32.1024, 22.2676)
  spline S165 degree 2 poles (32.1024, 22.2676) (32.4845, 22.2676) (32.7392, 22.0402) knots 0 0 0 1 1 1
  spline S166 degree 2 poles (32.7392, 22.0402) (33.0182, 21.7915) (33.0182, 21.37) knots 0 0 0 1 1 1
  spline S167 degree 2 poles (32.6694, 21.37) (32.6694, 21.6277) (32.3389, 21.9067) (32.1024, 21.9067) knots 0 0 0 1 2 2 2
  line L132 (32.1024, 21.9067) -> (31.0864, 21.9067)
  line L133 (31.0864, 21.9067) -> (31.0864, 20.8362)
  line L134 (31.0864, 20.8362) -> (32.2752, 20.8362)
  spline S168 degree 2 poles (32.2752, 20.8362) (32.3844, 20.8362) (32.5057, 20.9454) knots 0 0 0 1 1 1
  spline S169 degree 2 poles (32.5057, 20.9454) (32.6694, 21.097) (32.6694, 21.37) knots 0 0 0 1 1 1
  spline S170 degree 2 poles (35.9295, 20.6391) (35.9295, 19.9992) (35.6111, 19.5231) knots 0 0 0 1 1 1
  spline S171 degree 2 poles (35.6111, 19.5231) (35.2623, 19.0076) (34.7225, 19.0076) knots 0 0 0 1 1 1
  spline S172 degree 2 poles (34.7225, 19.0076) (34.1827, 19.0076) (33.834, 19.5292) knots 0 0 0 1 1 1
  spline S173 degree 2 poles (33.834, 19.5292) (33.5155, 20.0053) (33.5155, 20.6391) knots 0 0 0 1 1 1
  spline S174 degree 2 poles (33.5155, 20.6391) (33.5155, 21.2669) (33.84, 21.7491) knots 0 0 0 1 1 1
  spline S175 degree 2 poles (33.84, 21.7491) (34.1948, 22.2585) (34.7225, 22.2585) knots 0 0 0 1 1 1
  spline S176 degree 2 poles (34.7225, 22.2585) (35.2866, 22.2585) (35.6232, 21.743) knots 0 0 0 1 1 1
  spline S177 degree 2 poles (35.6232, 21.743) (35.9295, 21.276) (35.9295, 20.6391) knots 0 0 0 1 1 1
  spline S178 degree 2 poles (35.5807, 20.6391) (35.5807, 21.1365) (35.3776, 21.4852) knots 0 0 0 1 1 1
  spline S179 degree 2 poles (35.3776, 21.4852) (35.1471, 21.8976) (34.7225, 21.8976) knots 0 0 0 1 1 1
  spline S180 degree 2 poles (34.7225, 21.8976) (34.3222, 21.8976) (34.0796, 21.4852) knots 0 0 0 1 1 1
  spline S181 degree 2 poles (34.0796, 21.4852) (33.8643, 21.1274) (33.8643, 20.6391) knots 0 0 0 1 1 1
  spline S182 degree 2 poles (33.8643, 20.6391) (33.8643, 20.1387) (34.0735, 19.7809) knots 0 0 0 1 1 1
  spline S183 degree 2 poles (34.0735, 19.7809) (34.3101, 19.3685) (34.7225, 19.3685) knots 0 0 0 1 1 1
  spline S184 degree 2 poles (34.7225, 19.3685) (35.135, 19.3685) (35.3715, 19.7809) knots 0 0 0 1 1 1
  spline S185 degree 2 poles (35.3715, 19.7809) (35.5807, 20.1387) (35.5807, 20.6391) knots 0 0 0 1 1 1
  spline S186 degree 2 poles (38.8469, 21.37) (38.8469, 20.8878) (38.5284, 20.6422) knots 0 0 0 1 1 1
  spline S187 degree 2 poles (38.5284, 20.6422) (38.3161, 20.4754) (38.1069, 20.4754) knots 0 0 0 1 1 1
  line L135 (38.1069, 20.4754) -> (38.0129, 20.4784)
  line L136 (38.0129, 20.4784) -> (38.8135, 19.2926)
  spline S188 degree 2 poles (38.8135, 19.2926) (38.8469, 19.2381) (38.8469, 19.1865) knots 0 0 0 1 1 1
  spline S189 degree 2 poles (38.8469, 19.1865) (38.8469, 19.1107) (38.7377, 19.0015) (38.6679, 19.0015) knots 0 0 0 1 2 2 2
  spline S190 degree 2 poles (38.6679, 19.0015) (38.5861, 19.0015) (38.5345, 19.0773) knots 0 0 0 1 1 1
  line L137 (38.5345, 19.0773) -> (37.5823, 20.4754)
  line L138 (37.5823, 20.4754) -> (36.9151, 20.4754)
  line L139 (36.9151, 20.4754) -> (36.9151, 19.1865)
  spline S191 degree 2 poles (36.9151, 19.1865) (36.9151, 19.0015) (36.7422, 19.0015) knots 0 0 0 1 1 1
  spline S192 degree 2 poles (36.7422, 19.0015) (36.5663, 19.0015) (36.5663, 19.1865) knots 0 0 0 1 1 1
  line L140 (36.5663, 19.1865) -> (36.5663, 22.2676)
  line L141 (36.5663, 22.2676) -> (37.931, 22.2676)
  spline S193 degree 2 poles (37.931, 22.2676) (38.3131, 22.2676) (38.5679, 22.0402) knots 0 0 0 1 1 1
  spline S194 degree 2 poles (38.5679, 22.0402) (38.8469, 21.7915) (38.8469, 21.37) knots 0 0 0 1 1 1
  spline S195 degree 2 poles (38.4981, 21.37) (38.4981, 21.6277) (38.1676, 21.9067) (37.931, 21.9067) knots 0 0 0 1 2 2 2
  line L142 (37.931, 21.9067) -> (36.9151, 21.9067)
  line L143 (36.9151, 21.9067) -> (36.9151, 20.8362)
  line L144 (36.9151, 20.8362) -> (38.1039, 20.8362)
  spline S196 degree 2 poles (38.1039, 20.8362) (38.213, 20.8362) (38.3343, 20.9454) knots 0 0 0 1 1 1
  spline S197 degree 2 poles (38.3343, 20.9454) (38.4981, 21.097) (38.4981, 21.37) knots 0 0 0 1 1 1
  spline S198 degree 2 poles (44.3813, 21.1425) (44.3813, 20.069) (43.8173, 19.511) knots 0 0 0 1 1 1
  spline S199 degree 2 poles (43.8173, 19.511) (43.3533, 19.0591) (42.6922, 19.0591) knots 0 0 0 1 1 1
  line L145 (42.6922, 19.0591) -> (41.6763, 19.0591)
  line L146 (41.6763, 19.0591) -> (41.6763, 22.9894)
  line L147 (41.6763, 22.9894) -> (42.6861, 22.9894)
  spline S200 degree 2 poles (42.6861, 22.9894) (43.3412, 22.9894) (43.8173, 22.5588) knots 0 0 0 1 1 1
  spline S201 degree 2 poles (43.8173, 22.5588) (44.3813, 22.0493) (44.3813, 21.1425) knots 0 0 0 1 1 1
  spline S202 degree 2 poles (44.0265, 21.1456) (44.0265, 21.8643) (43.5807, 22.2767) knots 0 0 0 1 1 1
  spline S203 degree 2 poles (43.5807, 22.2767) (43.2017, 22.6194) (42.6861, 22.6194) knots 0 0 0 1 1 1
  line L148 (42.6861, 22.6194) -> (42.0311, 22.6194)
  line L149 (42.0311, 22.6194) -> (42.0311, 19.42)
  line L150 (42.0311, 19.42) -> (42.6922, 19.42)
  spline S204 degree 2 poles (42.6922, 19.42) (43.2199, 19.42) (43.5868, 19.8021) knots 0 0 0 1 1 1
  spline S205 degree 2 poles (43.5868, 19.8021) (44.0265, 20.2631) (44.0265, 21.1456) knots 0 0 0 1 1 1
  spline S206 degree 2 poles (47.4746, 20.6391) (47.4746, 19.9992) (47.1562, 19.5231) knots 0 0 0 1 1 1
  spline S207 degree 2 poles (47.1562, 19.5231) (46.8074, 19.0076) (46.2676, 19.0076) knots 0 0 0 1 1 1
  spline S208 degree 2 poles (46.2676, 19.0076) (45.7278, 19.0076) (45.3791, 19.5292) knots 0 0 0 1 1 1
  spline S209 degree 2 poles (45.3791, 19.5292) (45.0607, 20.0053) (45.0607, 20.6391) knots 0 0 0 1 1 1
  spline S210 degree 2 poles (45.0607, 20.6391) (45.0607, 21.2669) (45.3851, 21.7491) knots 0 0 0 1 1 1
  spline S211 degree 2 poles (45.3851, 21.7491) (45.74, 22.2585) (46.2676, 22.2585) knots 0 0 0 1 1 1
  spline S212 degree 2 poles (46.2676, 22.2585) (46.8317, 22.2585) (47.1683, 21.743) knots 0 0 0 1 1 1
  spline S213 degree 2 poles (47.1683, 21.743) (47.4746, 21.276) (47.4746, 20.6391) knots 0 0 0 1 1 1
  spline S214 degree 2 poles (47.1259, 20.6391) (47.1259, 21.1365) (46.9227, 21.4852) knots 0 0 0 1 1 1
  spline S215 degree 2 poles (46.9227, 21.4852) (46.6922, 21.8976) (46.2676, 21.8976) knots 0 0 0 1 1 1
  spline S216 degree 2 poles (46.2676, 21.8976) (45.8673, 21.8976) (45.6247, 21.4852) knots 0 0 0 1 1 1
  spline S217 degree 2 poles (45.6247, 21.4852) (45.4094, 21.1274) (45.4094, 20.6391) knots 0 0 0 1 1 1
  spline S218 degree 2 poles (45.4094, 20.6391) (45.4094, 20.1387) (45.6187, 19.7809) knots 0 0 0 1 1 1
  spline S219 degree 2 poles (45.6187, 19.7809) (45.8552, 19.3685) (46.2676, 19.3685) knots 0 0 0 1 1 1
  spline S220 degree 2 poles (46.2676, 19.3685) (46.6801, 19.3685) (46.9166, 19.7809) knots 0 0 0 1 1 1
  spline S221 degree 2 poles (46.9166, 19.7809) (47.1259, 20.1387) (47.1259, 20.6391) knots 0 0 0 1 1 1
  line L151 (51.1956, 22.0553) -> (50.6315, 19.1683)
  spline S222 degree 2 poles (50.6315, 19.1683) (50.5982, 19.0015) (50.4223, 19.0015) knots 0 0 0 1 1 1
  spline S223 degree 2 poles (50.4223, 19.0015) (50.2373, 19.0015) (50.1918, 19.1683) knots 0 0 0 1 1 1
  line L152 (50.1918, 19.1683) -> (49.5701, 21.4579)
  line L153 (49.5701, 21.4579) -> (48.9879, 19.1683)
  spline S224 degree 2 poles (48.9879, 19.1683) (48.9484, 19.0015) (48.7695, 19.0015) knots 0 0 0 1 1 1
  spline S225 degree 2 poles (48.7695, 19.0015) (48.5845, 19.0015) (48.5481, 19.1744) knots 0 0 0 1 1 1
  line L154 (48.5481, 19.1744) -> (47.9507, 22.0553)
  spline S226 degree 2 poles (47.9507, 22.0553) (47.9265, 22.1524) (48.0387, 22.2737) (48.1266, 22.2737) knots 0 0 0 1 2 2 2
  spline S227 degree 2 poles (48.1266, 22.2737) (48.2661, 22.2737) (48.2934, 22.1312) knots 0 0 0 1 1 1
  line L155 (48.2934, 22.1312) -> (48.7877, 19.7566)
  line L156 (48.7877, 19.7566) -> (49.3912, 22.1342)
  spline S228 degree 2 poles (49.3912, 22.1342) (49.4246, 22.2737) (49.5701, 22.2737) knots 0 0 0 1 1 1
  spline S229 degree 2 poles (49.5701, 22.2737) (49.7036, 22.2737) (49.74, 22.1524) knots 0 0 0 1 1 1
  line L157 (49.74, 22.1524) -> (50.3829, 19.7748)
  line L158 (50.3829, 19.7748) -> (50.8499, 22.1281)
  spline S230 degree 2 poles (50.8499, 22.1281) (50.8772, 22.2737) (51.0167, 22.2737) knots 0 0 0 1 1 1
  spline S231 degree 2 poles (51.0167, 22.2737) (51.1016, 22.2737) (51.2138, 22.1554) (51.1956, 22.0553) knots 0 0 0 1 2 2 2
  spline S232 degree 2 poles (54.116, 19.1895) (54.116, 19.0076) (53.9704, 19.0076) knots 0 0 0 1 1 1
  spline S233 degree 2 poles (53.9704, 19.0076) (53.8673, 19.0076) (53.7733, 19.141) knots 0 0 0 1 1 1
  line L159 (53.7733, 19.141) -> (52.0963, 21.5671)
  line L160 (52.0963, 21.5671) -> (52.0963, 19.1926)
  spline S234 degree 2 poles (52.0963, 19.1926) (52.0963, 19.0076) (51.9234, 19.0076) knots 0 0 0 1 1 1
  spline S235 degree 2 poles (51.9234, 19.0076) (51.7475, 19.0076) (51.7475, 19.1926) knots 0 0 0 1 1 1
  line L161 (51.7475, 19.1926) -> (51.7475, 22.113)
  spline S236 degree 2 poles (51.7475, 22.113) (51.7475, 22.2858) (51.9113, 22.2858) knots 0 0 0 1 1 1
  spline S237 degree 2 poles (51.9113, 22.2858) (52.0265, 22.2858) (52.1084, 22.1645) knots 0 0 0 1 1 1
  line L162 (52.1084, 22.1645) -> (53.7672, 19.7627)
  line L163 (53.7672, 19.7627) -> (53.7672, 22.0978)
  spline S238 degree 2 poles (53.7672, 22.0978) (53.7672, 22.2858) (53.9431, 22.2858) knots 0 0 0 1 1 1
  spline S239 degree 2 poles (53.9431, 22.2858) (54.116, 22.2858) (54.116, 22.1008) knots 0 0 0 1 1 1
  line L164 (54.116, 22.1008) -> (54.116, 19.1895)
  line L165 (58.7104, 20.4693) -> (57.2699, 20.4693)
  spline S240 degree 2 poles (57.2699, 20.4693) (57.091, 20.4693) (57.091, 20.6482) knots 0 0 0 1 1 1
  spline S241 degree 2 poles (57.091, 20.6482) (57.091, 20.8241) (57.2699, 20.8241) knots 0 0 0 1 1 1
  line L166 (57.2699, 20.8241) -> (58.7104, 20.8241)
  spline S242 degree 2 poles (58.7104, 20.8241) (58.8893, 20.8241) (58.8893, 20.6482) knots 0 0 0 1 1 1
  spline S243 degree 2 poles (58.8893, 20.6482) (58.8893, 20.4693) (58.7104, 20.4693) knots 0 0 0 1 1 1
  spline S244 degree 2 poles (64.7604, 20.9788) (64.7604, 20.166) (64.3783, 19.5989) knots 0 0 0 1 1 1
  spline S245 degree 2 poles (64.3783, 19.5989) (63.9598, 18.9773) (63.2805, 18.9773) knots 0 0 0 1 1 1
  spline S246 degree 2 poles (63.2805, 18.9773) (62.6073, 18.9773) (62.1766, 19.5989) knots 0 0 0 1 1 1
  spline S247 degree 2 poles (62.1766, 19.5989) (61.7763, 20.1782) (61.7763, 20.9788) knots 0 0 0 1 1 1
  spline S248 degree 2 poles (61.7763, 20.9788) (61.7763, 21.7854) (62.1524, 22.3798) knots 0 0 0 1 1 1
  spline S249 degree 2 poles (62.1524, 22.3798) (62.5648, 23.0227) (63.2168, 23.0227) knots 0 0 0 1 1 1
  spline S250 degree 2 poles (63.2168, 23.0227) (63.9143, 23.0227) (64.3541, 22.3798) knots 0 0 0 1 1 1
  spline S251 degree 2 poles (64.3541, 22.3798) (64.7604, 21.7854) (64.7604, 20.9788) knots 0 0 0 1 1 1
  spline S252 degree 2 poles (64.4056, 20.9788) (64.4056, 21.652) (64.1084, 22.1221) knots 0 0 0 1 1 1
  spline S253 degree 2 poles (64.1084, 22.1221) (63.7779, 22.6558) (63.2168, 22.6558) knots 0 0 0 1 1 1
  spline S254 degree 2 poles (63.2168, 22.6558) (62.6952, 22.6558) (62.398, 22.1221) knots 0 0 0 1 1 1
  spline S255 degree 2 poles (62.398, 22.1221) (62.1372, 21.6581) (62.1372, 20.9788) knots 0 0 0 1 1 1
  spline S256 degree 2 poles (62.1372, 20.9788) (62.1372, 20.3116) (62.4223, 19.8476) knots 0 0 0 1 1 1
  spline S257 degree 2 poles (62.4223, 19.8476) (62.7407, 19.3381) (63.2805, 19.3381) knots 0 0 0 1 1 1
  spline S258 degree 2 poles (63.2805, 19.3381) (63.8264, 19.3381) (64.1327, 19.8476) knots 0 0 0 1 1 1
  spline S259 degree 2 poles (64.1327, 19.8476) (64.4056, 20.3055) (64.4056, 20.9788) knots 0 0 0 1 1 1
  line L167 (67.9052, 19.0531) -> (65.4731, 19.0531)
  line L168 (65.4731, 19.0531) -> (65.4731, 22.8044)
  spline S260 degree 2 poles (65.4731, 22.8044) (65.4731, 22.9894) (65.652, 22.9894) knots 0 0 0 1 1 1
  spline S261 degree 2 poles (65.652, 22.9894) (65.8279, 22.9894) (65.8279, 22.8044) knots 0 0 0 1 1 1
  line L169 (65.8279, 22.8044) -> (65.8279, 19.4139)
  line L170 (65.8279, 19.4139) -> (67.9052, 19.4139)
  spline S262 degree 2 poles (67.9052, 19.4139) (68.0842, 19.4139) (68.0842, 19.235) knots 0 0 0 1 1 1
  spline S263 degree 2 poles (68.0842, 19.235) (68.0842, 19.0531) (67.9052, 19.0531) knots 0 0 0 1 1 1
  spline S264 degree 2 poles (71.4746, 21.1425) (71.4746, 20.069) (70.9105, 19.511) knots 0 0 0 1 1 1
  spline S265 degree 2 poles (70.9105, 19.511) (70.4466, 19.0591) (69.7854, 19.0591) knots 0 0 0 1 1 1
  line L171 (69.7854, 19.0591) -> (68.7695, 19.0591)
  line L172 (68.7695, 19.0591) -> (68.7695, 22.9894)
  line L173 (68.7695, 22.9894) -> (69.7794, 22.9894)
  spline S266 degree 2 poles (69.7794, 22.9894) (70.4344, 22.9894) (70.9105, 22.5588) knots 0 0 0 1 1 1
  spline S267 degree 2 poles (70.9105, 22.5588) (71.4746, 22.0493) (71.4746, 21.1425) knots 0 0 0 1 1 1
  spline S268 degree 2 poles (71.1198, 21.1456) (71.1198, 21.8643) (70.674, 22.2767) knots 0 0 0 1 1 1
  spline S269 degree 2 poles (70.674, 22.2767) (70.2949, 22.6194) (69.7794, 22.6194) knots 0 0 0 1 1 1
  line L174 (69.7794, 22.6194) -> (69.1243, 22.6194)
  line L175 (69.1243, 22.6194) -> (69.1243, 19.42)
  line L176 (69.1243, 19.42) -> (69.7854, 19.42)
  spline S270 degree 2 poles (69.7854, 19.42) (70.3131, 19.42) (70.6801, 19.8021) knots 0 0 0 1 1 1
  spline S271 degree 2 poles (70.6801, 19.8021) (71.1198, 20.2631) (71.1198, 21.1456) knots 0 0 0 1 1 1
  spline S272 degree 2 poles (77.0121, 21.9613) (77.0121, 21.5186) (76.7786, 21.2578) knots 0 0 0 1 1 1
  spline S273 degree 2 poles (76.7786, 21.2578) (76.536, 20.9788) (76.0993, 20.9788) knots 0 0 0 1 1 1
  line L177 (76.0993, 20.9788) -> (74.8347, 20.9788)